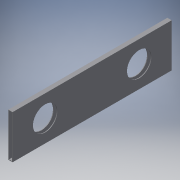
# Autodesk Inventor part: DRL SSS
Saved by Autodesk Inventor 2018.2 (Build 222227000, 227)
## iProperties
Created: 2018-01-13
Part Number: DRL SSS
Material: Generic
Document SubType Name: Modeling
Designer: Orangeracer
Density: 1 g/cm^3
Appearance: Default
Author: Orangeracer
Autodesk Inventor part; units mm, degrees
ref_plane "YZ Plane" through (0, 0, 0) normal (1, 0, 0) x (0, 1, 0)
ref_plane "XZ Plane" through (0, 0, 0) normal (0, 1, 0) x (-1, 0, 0)
ref_plane "XY Plane" through (0, 0, 0) normal (0, 0, 1) x (1, 0, 0)
sketch "Sketch1" plane through (0, 0, 0) normal (0, 0, 1) x (1, 0, 0)
  line L0 (0, 0) -> (-5.08, 0)
  line L1 (-5.08, 0) -> (-5.08, -50.8)
  line L2 (-5.08, -50.8) -> (0, -50.8)
  line L3 (0, -50.8) -> (0, 0)
  line L4 (-4.318, -0.762) -> (-0.762, -0.762)
  line L5 (-0.762, -0.762) -> (-0.762, -50.038)
  line L6 (-0.762, -50.038) -> (-4.318, -50.038)
  line L7 (-4.318, -50.038) -> (-4.318, -0.762)
  dimension "d0" = 5.08
  dimension "d1" = 50.8
  dimension "d2" = 0.762
  constraints: 16 end point, 4 parallel, 2 perpendicular, 1 horizontal, 3 other
  measures "d0" distance of L2.end L1.end
  measures "d1" distance of L1.end L0.end
  measures "d2" distance between parallel lines of L0 L4
extrude "Extrusion1" add sketch "Sketch1" along normal blind 186.2252
sketch "Sketch2" plane through (0, -50.8, 0) normal (1, 0, 0) x (0, 0, -1)
  circle A0 centre (-148.1252, 25.4) radius 14.2875
  circle A1 centre (-38.1, 25.4) radius 14.2875
  line L0 (0, 0) -> (-186.2252, 0) projected
  line L1 (0, 0) -> (0, 50.8) projected
  line L2 (-186.2252, 0) -> (-186.2252, 50.8) projected
  line L3 (0, 50.8) -> (-186.2252, 50.8) projected
  dimension "d5" = 25.4
  dimension "d6" = 38.1
  dimension "d7" = 28.575
  dimension "d8" = 38.1
  dimension "d9" = 25.4
  dimension "d10" = 28.575
  dimension "d13" = 110.0252
  constraints: 2 centre point
  measures "d5" distance from line of L0 A1.centre
  measures "d6" distance from line of L1 A1.centre
  measures "d7" diameter of A1
  measures "d8" distance from line of L2 A0.centre
  measures "d9" distance from line of L3 A0.centre
  measures "d10" diameter of A0
  measures "d13" distance of A1.centre A0.centre
extrude "Extrusion2" cut sketch "Sketch2" against normal blind 198.12 contours A0 | A1
body "Solid1"
